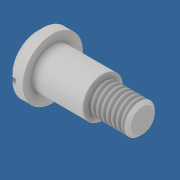
# Autodesk Inventor part: Zapfen
Saved by Autodesk Inventor 2018 (Build 220112000, 112)
## iProperties
Created: 2018-10-20
Part Number: Zapfen
Material: Generisch
Document SubType Name: Modeling
Designer: M.Knabel
Density: 1 g/cm^3
Appearance: Vorgabe
Author: M.Knabel
Autodesk Inventor part; units mm, degrees
ref_plane "YZ Plane" through (0, 0, 0) normal (1, 0, 0) x (0, 1, 0)
ref_plane "XZ Plane" through (0, 0, 0) normal (0, 1, 0) x (-1, 0, 0)
ref_plane "XY Plane" through (0, 0, 0) normal (0, 0, 1) x (1, 0, 0)
sketch "Skizze1" plane through (0, 0, 0) normal (0, 0, 1) x (1, 0, 0)
  line L0 (-2.1, 0) -> (12.6, 0) projected
  line L1 (0, -0.6) -> (0, 3.6) projected
  line L2 (0, 0) -> (0, 3)
  line L3 (0, 3) -> (1.5, 3)
  line L4 (1.5, 3) -> (1.5, 2)
  line L5 (1.5, 2) -> (6.5, 2)
  line L6 (6.5, 2) -> (6.5, 1.5)
  line L7 (6.5, 1.5) -> (10.5, 1.5)
  line L8 (10.5, 1.5) -> (10.5, 0)
  line L9 (10.5, 0) -> (0, 0)
  dimension "d0" = 6
  dimension "d1" = 4
  dimension "d2" = 3
  dimension "d3" = 10.5
  dimension "d4" = 4
  dimension "d5" = 9
  constraints: 16 end point, 4 perpendicular, 2 horizontal, 2 point on line, 1 collinear
  measures "d0" diameter of L3 L0
  measures "d1" diameter of L5 L0
  measures "d2" diameter of L7 L0
  measures "d3" distance between parallel lines of L8 L1
  measures "d4" distance between parallel lines of L6 L8
  measures "d5" distance between parallel lines of L4 L8
revolve "Umdrehung1" add sketch "Skizze1" angle 360 about axis through (-10, 0, 0) along (1, 0, 0)
thread "Gewinde1" size "M3x0.5" class "6g" standard "ANSI Metric M Profile" full length
chamfer "Fase1" distance 0.3 angle 45 1 edges at (10.5, -1.5, 0)
chamfer "Fase2" distance 0.5 angle 45 1 edges at (0, -3, 0)
sketch "Skizze2" plane through (0, 0, 0) normal (-1, 0, 0) x (0, 0, 1)
  line L0 (0, -4.2) -> (0, 4.2) projected
  line L1 (-4.2, 0) -> (4.2, 0) projected
  circle A0 centre (0, 0) radius 3 projected
  circle A1 centre (0, 0) radius 3 projected
  line L2 (-0.25, 2.9896) -> (-0.25, -2.9896)
  line L3 (0.25, -2.9896) -> (0.25, 2.9896)
  arc A2 (-0.25, -2.9896) -> (0.25, -2.9896) centre (0, 0) ccw
  arc A3 (0.25, 2.9896) -> (-0.25, 2.9896) centre (0, 0) ccw
  dimension "d15" = 0.5
  constraints: 8 point on circle, 4 end point, 2 centre point, 1 coincident, 1 parallel, 1 vertical, 1 other
  measures "d15" distance between parallel lines of L3 L2
extrude "Extrusion1" cut sketch "Skizze2" against normal blind 0.8 contours A0 L2 L1 L0 | L0 L1 L3 A0 | L1 L2 A0 L0 | L0 A0 L3 L1
